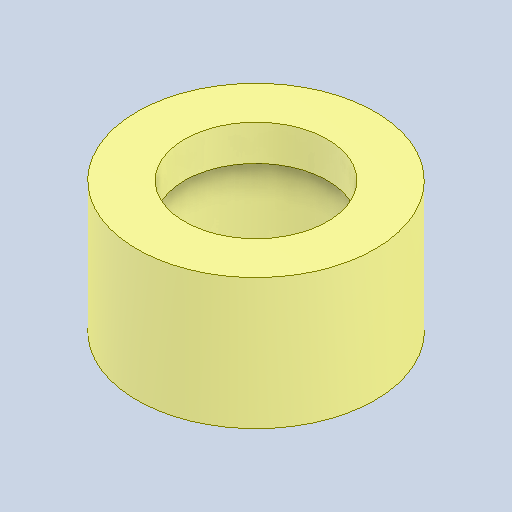
# Autodesk Inventor part: TransmissionBeltTensionerRoller
Saved by Autodesk Inventor 2023 (Build 270158000, 158)
## iProperties
Created: 2019-05-28
Part Number: TransmissionBeltTensionerRoller
Material: Generic
Document SubType Name: Modeling
Designer: Jochen
Density: 1 g/cm^3
Appearance: Default
Sending System: SolidWorks 2017
Last Author: Felix
Last Saved: 2020-09-07
Author: Jochen
Autodesk Inventor part; units mm, degrees
ref_plane "YZ Plane" through (0, 0, 0) normal (1, 0, 0) x (0, 1, 0)
ref_plane "XZ Plane" through (0, 0, 0) normal (0, 1, 0) x (-1, 0, 0)
ref_plane "XY Plane" through (0, 0, 0) normal (0, 0, 1) x (1, 0, 0)
sketch "Sketch1" plane through (0, 0, 0) normal (0, 1, 0) x (-1, 0, 0)
  circle A0 centre (0, 0) radius 3
  circle A1 centre (0, 0) radius 5
  circle A2 centre (0, 0) radius 3.65
  dimension "d0" = 6
  dimension "d1" = 10
  dimension "d2" = 7.3
  constraints: 3 centre point, 3 coincident
  measures "d0" diameter of A0
  measures "d1" diameter of A1
  measures "d2" diameter of A2
extrude "Extrusion1" add sketch "Sketch1" along normal blind 4 contours A1
extrude "Extrusion2" add sketch "Sketch1" along normal blind 1.5 from surface at 4 contours A1 | A2
chamfer "Chamfer1" distance 0.5 angle 45 1 edges at (3.65, 0, 0)
body "Solid1"
